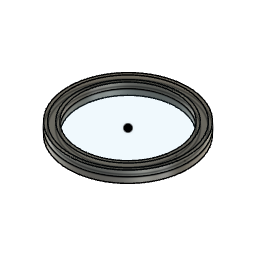
Enclosure v49 (Autodesk Fusion 360 archive; units mm, degrees)
design "Ball Bearing"
Autodesk Fusion 360 part; units mm, degrees
sketch "Sketch1" plane through (0, 0, 0) normal (0, 0, 1) x (1, 0, 0)
  circle A0 centre (0, 0) radius 25.125
  circle A1 centre (0, 0) radius 26.625
  circle A2 centre (0, 0) radius 31.125
  circle A3 centre (0, 0) radius 29.625
  dimension "d1" = 50.25
  dimension "d2" = 62.25
  dimension "d3" = 53.25
  dimension "d4" = 59.25
  constraint coincident A0.centre A1.centre
  constraint concentric A1 A2
  constraint concentric A1 A3
  measures "d1" diameter of A0
  measures "d2" diameter of A2
  measures "d3" diameter of A1
  measures "d4" diameter of A3
extrude "Extrude1" add sketch "Sketch1" along normal mid plane 6 contours A1 makes body 1
extrude "Extrude2" add sketch "Sketch1" along normal mid plane 6 separate body contours A3 makes body 2
extrude "Extrude3" add sketch "Sketch1" along normal mid plane 6 separate body contours A2 makes body 3

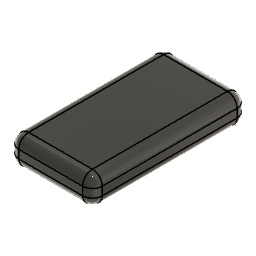
design "3.7 V Li-Ion Battery"
Autodesk Fusion 360 part; units mm, degrees
sketch "Sketch1" plane through (0, 0, 0) normal (0, 0, 1) x (1, 0, 0)
  line L0 (8.5, 15.75) -> (-8.5, 15.75)
  line L1 (-8.5, 15.75) -> (-8.5, -15.75)
  line L2 (-8.5, -15.75) -> (8.5, -15.75)
  line L3 (8.5, -15.75) -> (8.5, 15.75)
  line L4 (8.5, 15.75) -> (-8.5, -15.75) construction
  line L5 (-8.5, 15.75) -> (8.5, -15.75) construction
  dimension "d1" = 31.5
  dimension "d2" = 17
  constraint horizontal L0
  constraint perpendicular L0 L1
  constraint parallel L0 L2
  constraint parallel L1 L3
  constraint coincident L4 origin
  constraint coincident L5 origin
  measures "d1" distance of L0.end L1.end
  measures "d2" distance of L0.start L0.end
extrude "Extrude1" add sketch "Sketch1" along normal blind 5.7
fillet "Fillet1" radius 2 12 edges at (0, -15.75, 5.7) (-8.5, 0, 5.7) (-8.5, -15.75, 2.85) (8.5, -15.75, 2.85) (8.5, 0, 5.7) (8.5, 15.75, 2.85) (-8.5, 15.75, 2.85) (0, 15.75, 5.7) (0, 15.75, 0) (-8.5, 0, 0) (8.5, 0, 0) (0, -15.75, 0)
